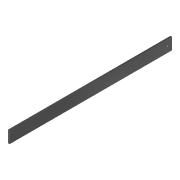
# Autodesk Inventor part: LIVER
Saved by Autodesk Inventor 2014 (Build 180170000, 170)
## iProperties
Created: 2014-12-19
Part Number: LIVER
Material: Steel, Mild
Document SubType Name: Modeling
Designer: Ebrahim
Density: 7.86 g/cm^3
Appearance: Steel - Polished
Mass: 200.263 g
Surface Area: 192.041 cm^2
Volume: 25.4788 cm^3
Author: Ebrahim
Autodesk Inventor part; units mm, degrees
ref_plane "YZ Plane" through (0, 0, 0) normal (1, 0, 0) x (0, 1, 0)
ref_plane "XZ Plane" through (0, 0, 0) normal (0, 1, 0) x (-1, 0, 0)
ref_plane "XY Plane" through (0, 0, 0) normal (0, 0, 1) x (1, 0, 0)
sketch "Sketch1" plane through (0, 0, 0) normal (0, 1, 0) x (-1, 0, 0)
  line L0 (-331, 12.5) -> (9, 12.5)
  line L1 (9, 12.5) -> (9, -12.5)
  line L2 (9, -12.5) -> (-331, -12.5)
  line L3 (-331, -12.5) -> (-331, 12.5)
  line L4 (-399, 0) -> (77, 0) construction
  point P0 (0, 0)
  point P1 (9, 0)
  dimension "d0" = 340
  dimension "d1" = 25
  dimension "d2" = 9
  constraints: 8 end point, 2 parallel, 1 horizontal, 1 midpoint, 1 perpendicular, 1 point on line
  measures "d0" distance of L0.start L0.end
  measures "d1" distance of L2.end L0.start
  measures "d2" distance from line of L1 point (0, 0)
extrude "Extrusion1" add sketch "Sketch1" against normal blind 3
hole "Hole1" at (0, 0, 0) direction (0, -1, 0) diameter 3 end through all
body "Solid1"
